8mm tooling v1 (Autodesk Fusion 360 design; units mm, degrees)
Autodesk Fusion 360 part; units mm, degrees
sketch "Sketch1" plane through (0, 0, 0) normal (0, 1, 0) x (1, 0, 0)
  line L0 (0, 0) -> (144, 0)
  line L1 (144, -40) -> (0, -40)
  line L2 (0, -40) -> (0, 0)
  line L3 (0, -20) -> (144, -20)
  line L4 (0, 0) -> (10, 0)
  line L5 (144, 0) -> (140, 0)
  line L6 (10, 0) -> (36, 0)
  line L7 (36, -40) -> (62, -40)
  line L8 (62, 0) -> (88, 0)
  line L9 (88, -40) -> (114, -40)
  line L10 (114, 0) -> (140, 0)
  circle A0 centre (9.5, -30) radius 4
  line L11 (134, -20) -> (144, -20)
  line L12 (144, -40) -> (144, 0)
  line L13 (0, 0) -> (144, 0)
  line L14 (144, 0) -> (144, -5)
  line L15 (144, -5) -> (0, -5)
  line L16 (0, -5) -> (0, 0)
  line L17 (0, -40) -> (5, -40)
  line L18 (5, -40) -> (5, 0)
  line L19 (5, 0) -> (0, 0)
  line L20 (0, 0) -> (0, -40)
  line L21 (144, -40) -> (139, -40)
  line L22 (139, -40) -> (139, 0)
  line L23 (139, 0) -> (144, 0)
  line L24 (144, 0) -> (144, -40)
  circle A1 centre (27.3571, -30) radius 4
  circle A2 centre (45.2143, -30) radius 4
  circle A3 centre (63.0714, -30) radius 4
  circle A4 centre (80.9286, -30) radius 4
  circle A5 centre (98.7857, -30) radius 4
  circle A6 centre (116.6429, -30) radius 4
  circle A7 centre (134.5, -30) radius 4
  circle A8 centre (9.5, -15) radius 4
  circle A9 centre (27.3571, -15) radius 4
  circle A10 centre (45.2143, -15) radius 4
  circle A11 centre (63.0714, -15) radius 4
  circle A12 centre (80.9286, -15) radius 4
  circle A13 centre (98.7857, -15) radius 4
  circle A14 centre (116.6429, -15) radius 4
  circle A15 centre (134.5, -15) radius 4
  dimension "d8" = 8
  dimension "d16" = 5
  dimension "d17" = 5
  dimension "d75" = 125
  dimension "d76" = 15
  constraint horizontal L0
  constraint horizontal L1
  constraint vertical L2
  constraint coincident L0.start L2.end
  constraint midpoint L2 L3.start
  constraint coincident L0 L4.end
  constraint perpendicular L2 L4
  constraint coincident L0 L5.end
  constraint coincident L1 L7.start
  constraint coincident L0 L8.start
  constraint coincident L1 L9.start
  constraint coincident L0 L10.start
  constraint coincident L3 L11.start
  constraint coincident L1 L12.start
  constraint vertical L12
  constraint horizontal L13
  constraint vertical L14
  constraint horizontal L15
  constraint vertical L16
  constraint horizontal L17
  constraint vertical L18
  constraint horizontal L19
  constraint vertical L20
  constraint midpoint L4 L18.end
  constraint horizontal L21
  constraint vertical L22
  constraint horizontal L23
  constraint vertical L24
  measures "d8" diameter of A0
  measures "d16" distance of L0.start L15.end
  measures "d17" distance of L1.start L21.end
extrude "Extrude1" add sketch "Sketch1" along normal blind 5 contours L0 L2 L4 L13 L15 L16 L18 L19 L20 | L0 L4 L6 L8 L10 L13 L15 L18 L22 | L2 L3 L15 L18 L20 | L3 L11 L15 L18 L22 | L1 L2 L3 L17 L18 L20 | L0 L5 L10 L12 L13 L14 L15 L22 L23 L24 | L3 L11 L12 L15 L22 L24 | L1 L3 L7 L9 L11 L18 L22 | L1 L3 L11 L12 L21 L22 L24 | A1 | A2 | A3 | A4 | A5 | A6 | A7 | A8 | A9 | A10 | A11 | A12 | A13 | A14 | A15 makes body 1
fillet "Fillet2" radius 2 2 edges at (72, 5, 40) (72, 0, 40) on bodies 1
sketch "Sketch2" plane through (0, 0, 0) normal (0, -1, 0) x (1, 0, 0)
  line L0 (144, 38) -> (0, 38)
  line L1 (0, 38) -> (0, 0)
  line L2 (0, 0) -> (144, 0)
  line L3 (144, 0) -> (144, 38)
  line L4 (0, 0) -> (144, 0)
  line L5 (144, 0) -> (144, 5)
  line L6 (144, 5) -> (0, 5)
  line L7 (0, 5) -> (0, 0)
  line L8 (0, 0) -> (5, 0)
  line L9 (5, 0) -> (5, 38)
  line L10 (5, 38) -> (0, 38)
  line L11 (0, 38) -> (0, 0)
  line L12 (144, 0) -> (139, 0)
  line L13 (139, 0) -> (139, 38)
  line L14 (139, 38) -> (144, 38)
  line L15 (144, 38) -> (144, 0)
  circle A0 centre (9.5, 30) radius 4
  dimension "d22" = 5
  dimension "d23" = 5
  dimension "d24" = 5
  constraint horizontal L4
  constraint vertical L5
  constraint horizontal L6
  constraint vertical L7
  constraint coincident L1.end L2.start
  constraint horizontal L8
  constraint vertical L9
  constraint horizontal L10
  constraint vertical L11
  constraint horizontal L12
  constraint vertical L13
  constraint horizontal L14
  constraint vertical L15
  measures "d22" distance of L1.end L6.end
  measures "d23" distance of L1.end L8.end
  measures "d24" distance of L2.end L12.end
extrude "Extrude2" add sketch "Sketch2" along normal blind 5 contours L0 L3 L6 L13 L14 L15 | L2 L3 L4 L5 L6 L12 L13 L15 | L0 L1 L6 L9 L10 L11 | L2 L4 L6 L9 L13 | L1 L2 L4 L6 L7 L8 L9 L11 bodies 1
sketch "Sketch3" plane through (0, -5, 0) normal (0, -1, 0) x (1, 0, 0)
  line L0 (139, 38) -> (139, 5)
  line L1 (139, 5) -> (5, 5)
  line L2 (5, 5) -> (5, 38)
  line L3 (0, 38) -> (0, 0)
  line L4 (0, 0) -> (144, 0)
  line L5 (144, 0) -> (144, 38)
  line L6 (72, 0) -> (72, 5)
  line L7 (72, 5) -> (82, 5)
  line L8 (82, 5) -> (82, 0)
  line L9 (82, 0) -> (72, 0)
  line L10 (72, 0) -> (72, 5)
  line L11 (72, 0) -> (62, 0)
  line L12 (62, 0) -> (62, 5)
  line L13 (62, 5) -> (72, 5)
  line L14 (72, 5) -> (72, 0)
  line L15 (5, 5) -> (25, 5)
  line L16 (25, 5) -> (25, 0)
  line L17 (25, 0) -> (5, 0)
  line L18 (5, 0) -> (5, 5)
  line L19 (139, 5) -> (119, 5)
  line L20 (119, 5) -> (119, 0)
  line L21 (119, 0) -> (139, 0)
  line L22 (139, 0) -> (139, 5)
  line L23 (5, 38) -> (0, 38)
  line L24 (144, 38) -> (139, 38)
  dimension "d28" = 10
  dimension "d29" = 10
  dimension "d30" = 20
  dimension "d31" = 20
  constraint midpoint L4 L6.start
  constraint midpoint L1 L6.end
  constraint horizontal L7
  constraint vertical L8
  constraint horizontal L9
  constraint vertical L10
  constraint horizontal L11
  constraint vertical L12
  constraint horizontal L13
  constraint vertical L14
  constraint horizontal L15
  constraint vertical L16
  constraint horizontal L17
  constraint vertical L18
  constraint coincident L1.end L2.start
  constraint horizontal L19
  constraint vertical L20
  constraint horizontal L21
  constraint vertical L22
  constraint coincident L0.end L1.start
  measures "d28" distance of L6.end L7.end
  measures "d29" distance of L6.start L11.end
  measures "d30" distance of L1.end L15.end
  measures "d31" distance of L0.end L19.end
extrude "Extrude3" add sketch "Sketch3" along normal blind 10 contours L1 L4 L19 L20 L21 L22 | L1 L4 L6 L7 L8 L9 L10 L14 | L1 L4 L6 L10 L11 L12 L13 L14 | L1 L4 L15 L16 L17 L18 bodies 1
fillet "Fillet4" radius 10 6 edges at (5, -15, 2.5) (25, -15, 2.5) (62, -15, 2.5) (82, -15, 2.5) (119, -15, 2.5) (139, -15, 2.5) on bodies 1
sketch "Sketch4" plane through (0, 0, 5) normal (0, 0, 1) x (1, 0, 0)
  arc A0 (119, -5) -> (139, -5) centre (129, -5) ccw
  line L0 (139, -5) -> (139, 0)
  line L1 (139, 0) -> (5, 0)
  line L2 (5, 0) -> (5, -5)
  arc A1 (5, -5) -> (25, -5) centre (15, -5) ccw
  line L3 (25, -5) -> (62, -5)
  arc A2 (62, -5) -> (82, -5) centre (72, -5) ccw
  line L4 (82, -5) -> (119, -5)
  line L5 (15, -15) -> (15, 0)
  line L6 (72, -15) -> (72, 0)
  line L7 (129, -15) -> (129, 0)
  line L8 (5, -5) -> (139, -5)
  circle A3 centre (15, -5) radius 1.5
  circle A4 centre (10, -5) radius 1.5
  circle A5 centre (20, -5) radius 1.5
  circle A6 centre (72, -5) radius 1.5
  line L9 (62, -5) -> (82, -5)
  line L10 (62, -5) -> (67, -5)
  line L11 (82, -5) -> (77, -5)
  circle A7 centre (67, -5) radius 1.5
  circle A8 centre (77, -5) radius 1.5
  line L12 (119, -5) -> (139, -5)
  circle A9 centre (129, -5) radius 1.5
  line L13 (119, -5) -> (129, -5)
  circle A10 centre (124, -5) radius 1.5
  line L14 (139, -5) -> (129, -5)
  circle A11 centre (134, -5) radius 1.5
  line L15 (72, -5) -> (72, -15)
  circle A12 centre (72, -10) radius 1.5
  line L16 (15, -15) -> (15, -5)
  circle A13 centre (15, -10) radius 1.5
  line L17 (129, -15) -> (129, -5)
  circle A14 centre (129, -10) radius 1.5
  circle A15 centre (15, 0) radius 1.5
  circle A16 centre (72, 0) radius 1.5
  circle A17 centre (129, 0) radius 1.5
  dimension "d35" = 3
  dimension "d36" = 3
  dimension "d37" = 3
  dimension "d38" = 3
  dimension "d39" = 5
  dimension "d40" = 3
  dimension "d41" = 3
  dimension "d42" = 3
  dimension "d43" = 3
  dimension "d44" = 3
  dimension "d45" = 3
  dimension "d46" = 3
  dimension "d47" = 3
  dimension "d48" = 3
  dimension "d49" = 3
  dimension "d50" = 3
  constraint midpoint A1 L5.start
  constraint coincident L1 L5.end
  constraint midpoint A2 L6.start
  constraint midpoint L1 L6.end
  constraint midpoint A0 L7.start
  constraint coincident L1 L7.end
  constraint vertical L7
  constraint coincident L2.end A1.start
  constraint coincident A0.end L0.start
  constraint concentric A1 A3
  constraint coincident L8 A4.centre
  constraint concentric A2 A6
  constraint coincident L3.end A2.start
  constraint coincident A2.end L4.start
  constraint coincident L9 L10.end
  constraint perpendicular L6 L10
  constraint coincident L10.end A7.centre
  constraint coincident L11.end A8.centre
  constraint coincident A0.start L4.end
  constraint concentric A0 A9
  constraint coincident A0.centre A9.centre
  constraint midpoint L13 A10.centre
  constraint midpoint L14 A11.centre
  constraint coincident A2.centre A6.centre
  constraint midpoint L15 A12.centre
  constraint coincident A1.centre A3.centre
  constraint midpoint L16 A13.centre
  constraint midpoint L17 A14.centre
  constraint coincident L5.end A15.centre
  constraint coincident L6.end A16.centre
  constraint coincident L7.end A17.centre
  measures "d35" diameter of A3
  measures "d36" diameter of A4
  measures "d37" diameter of A5
  measures "d38" diameter of A6
  measures "d39" distance of A2.end L11.end
  measures "d40" diameter of A7
  measures "d41" diameter of A8
  measures "d42" diameter of A9
  measures "d43" diameter of A10
  measures "d44" diameter of A11
  measures "d45" diameter of A12
  measures "d46" diameter of A13
  measures "d47" diameter of A14
  measures "d48" diameter of A15
  measures "d49" diameter of A16
  measures "d50" diameter of A17
extrude "Extrude4" cut sketch "Sketch4" along normal blind 20 contours L8 L12 L13 A10 | L8 L12 L13 A10 | L7 L17 A14 | L7 L17 A14 | L8 L9 L11 A8 | L8 L9 L11 A8 | L8 L12 L14 A11 | L8 L12 L14 A11 | L6 L15 A12 | L6 L15 A12 | L7 L8 L12 A9 L13 | L7 L8 L12 A9 L13 L17 | L1 L7 A17 | L1 A17 | L7 L8 L12 A9 L14 L17 | L8 L9 L10 A7 | L8 L9 L10 A7 | L6 L8 A6 L9 L15 | L6 L8 A6 L9 | L7 L8 L12 A9 L14 | L1 L7 A17 | L8 A5 | L8 A5 | L6 L8 A6 L9 L15 | L6 L8 A6 L9 | L1 L6 A16 | L1 A16 | L5 L16 A13 | L5 L16 A13 | L1 L6 A16 | L8 A4 | L8 A4 | L5 L8 A3 L16 | L5 L8 A3 | L1 L5 A15 | L1 A15 | L1 L5 A15 | L5 L8 A3 L16 | L5 L8 A3 bodies 1
extrude "Extrude5" cut sketch "Sketch4" against normal blind 10 contours L8 L12 L13 A10 | L8 L12 L13 A10 | L7 L17 A14 | L7 L17 A14 | L8 L9 L11 A8 | L8 L9 L11 A8 | L8 L12 L14 A11 | L8 L12 L14 A11 | L6 L15 A12 | L6 L15 A12 | L7 L8 L12 A9 L13 | L7 L8 L12 A9 L13 L17 | L1 L7 A17 | L1 A17 | L7 L8 L12 A9 L14 L17 | L8 L9 L10 A7 | L8 L9 L10 A7 | L6 L8 A6 L9 L15 | L6 L8 A6 L9 | L7 L8 L12 A9 L14 | L1 L7 A17 | L8 A5 | L8 A5 | L6 L8 A6 L9 L15 | L6 L8 A6 L9 | L1 L6 A16 | L1 A16 | L5 L16 A13 | L5 L16 A13 | L1 L6 A16 | L8 A4 | L8 A4 | L5 L8 A3 L16 | L5 L8 A3 | L1 L5 A15 | L1 A15 | L1 L5 A15 | L5 L8 A3 L16 | L5 L8 A3 bodies 1
sketch "Sketch5" plane through (0, 0, 0) normal (0, 0, -1) x (-1, 0, 0)
  arc A0 (-139, -5) -> (-119, -5) centre (-129, -5) ccw
  line L0 (-119, -5) -> (-82, -5)
  arc A1 (-82, -5) -> (-62, -5) centre (-72, -5) ccw
  line L1 (-62, -5) -> (-25, -5)
  arc A2 (-25, -5) -> (-5, -5) centre (-15, -5) ccw
  line L2 (-5, -5) -> (0, -5)
  line L3 (0, -5) -> (0, 5)
  line L4 (0, 5) -> (-144, 5)
  line L5 (-144, 5) -> (-144, -5)
  line L6 (-144, -5) -> (-139, -5)
  circle A3 centre (-15, -10) radius 1.5
  circle A4 centre (-72, -5) radius 1.5
  circle A5 centre (-129, -5) radius 1.5
  circle A6 centre (-15, 0) radius 1.5
  circle A7 centre (-124, -5) radius 1.5
  circle A8 centre (-67, -5) radius 1.5
  circle A9 centre (-10, -5) radius 1.5
  circle A10 centre (-15, -5) radius 1.5
  circle A11 centre (-72, -10) radius 1.5
  circle A12 centre (-129, -10) radius 1.5
  circle A13 centre (-72, 0) radius 1.5
  circle A14 centre (-129, 0) radius 1.5
  circle A15 centre (-134, -5) radius 1.5
  circle A16 centre (-77, -5) radius 1.5
  circle A17 centre (-20, -5) radius 1.5
sketch "Sketch6" plane through (0, 0, 5) normal (0, 0, 1) x (1, 0, 0)
  circle A0 centre (72, 0) radius 3
  circle A1 centre (67, -5) radius 3
  circle A2 centre (77, -5) radius 3
  circle A3 centre (72, -10) radius 3
  circle A4 centre (15, 0) radius 3
  circle A5 centre (10, -5) radius 3
  circle A6 centre (20, -5) radius 3
  circle A7 centre (15, -10) radius 3
  circle A8 centre (129, 0) radius 3
  circle A9 centre (124, -5) radius 3
  circle A10 centre (134, -5) radius 3
  circle A11 centre (129, -10) radius 3
  point P0 (72, 0)
  point P1 (67, -5)
  point P2 (77, -5)
  point P3 (72, -10)
  point P4 (15, 0)
  point P5 (10, -5)
  point P6 (15, -10)
  point P7 (129, 0)
  point P8 (124, -5)
  point P9 (134, -5)
  point P10 (129, -10)
  dimension "d55" = 6
  dimension "d56" = 6
  dimension "d57" = 6
  dimension "d58" = 6
  dimension "d59" = 6
  dimension "d60" = 6
  dimension "d61" = 6
  dimension "d62" = 6
  dimension "d63" = 6
  dimension "d64" = 6
  dimension "d65" = 6
  dimension "d66" = 6
  constraint coincident P0 A0.centre
  constraint coincident P1 A1.centre
  constraint coincident P2 A2.centre
  constraint coincident P3 A3.centre
  constraint coincident P4 A4.centre
  constraint coincident P5 A5.centre
  constraint coincident P6 A7.centre
  constraint coincident P7 A8.centre
  constraint coincident P8 A9.centre
  constraint coincident P9 A10.centre
  constraint coincident P10 A11.centre
  measures "d55" diameter of A0
  measures "d56" diameter of A1
  measures "d57" diameter of A2
  measures "d58" diameter of A3
  measures "d59" diameter of A4
  measures "d60" diameter of A5
  measures "d61" diameter of A6
  measures "d62" diameter of A7
  measures "d63" diameter of A8
  measures "d64" diameter of A9
  measures "d65" diameter of A10
  measures "d66" diameter of A11
chamfer "Chamfer1" distance 3 angle 45 3 edges at (13.6015, -4.4576, 5) (70.6015, -4.4576, 5) (127.6015, -4.4576, 5) on bodies 1
extrude "Extrude6" cut sketch "Sketch6" along normal blind 20 bodies 1
extrude "Extrude7" cut sketch "Sketch6" against normal blind 3.5 bodies 1
fillet "Fillet5" radius 2 3 edges at (15, -15, 5) (72, -15, 5) (129, -15, 5) on bodies 1
extrude "Extrude8" cut sketch "Sketch1" along normal blind 10 contours A1 | A2 | A3 | A4 | A5 | A6 | A7 | A8 | A9 | A10 | A11 | A12 | A13 | A14 | A15 bodies 1
fillet "Fillet7" radius 3 16 edges at (130.7707, 5, 28.5535) (130.7707, 5, 13.5535) (112.9135, 5, 28.5535) (112.9135, 5, 13.5535) (95.0564, 5, 28.5535) (95.0564, 5, 13.5535) (77.1993, 5, 28.5535) (77.1993, 5, 13.5535) (59.3421, 5, 28.5535) (59.3421, 5, 13.5535) (41.485, 5, 28.5535) (41.485, 5, 13.5535) (23.6278, 5, 28.5535) (23.6278, 5, 13.5535) (5.7707, 5, 13.5535) (5.7707, 5, 28.5535) on bodies 1
sketch "Sketch7" plane through (0, 0, 0) normal (0, -1, 0) x (1, 0, 0)
  circle A0 centre (9.5, 30) radius 4
  arc A1 (132, 11.8775) -> (132, 18.1225) centre (134.5, 15) ccw
  line L0 (132, 11.8775) -> (132, 5)
  line L1 (132, 5) -> (139, 5)
  line L2 (139, 5) -> (139, 38)
  line L3 (139, 38) -> (5, 38)
  line L4 (5, 38) -> (5, 5)
  line L5 (5, 5) -> (12, 5)
  line L6 (12, 5) -> (12, 11.8775)
  arc A2 (12, 18.1225) -> (12, 11.8775) centre (9.5, 15) ccw
  line L7 (12, 18.1225) -> (12, 25)
  line L8 (12, 25) -> (18, 25)
  line L9 (18, 25) -> (18, 5)
  line L10 (18, 5) -> (69, 5)
  line L11 (69, 5) -> (69, 25)
  line L12 (69, 25) -> (75, 25)
  line L13 (75, 25) -> (75, 5)
  line L14 (75, 5) -> (126, 5)
  line L15 (126, 5) -> (126, 25)
  line L16 (126, 25) -> (132, 25)
  line L17 (132, 25) -> (132, 18.1225)
  circle A3 centre (80.9286, 15) radius 4
  circle A4 centre (134.5, 30) radius 4
  circle A5 centre (63.0714, 30) radius 4
  circle A6 centre (45.2143, 30) radius 4
  circle A7 centre (116.6429, 30) radius 4
  circle A8 centre (98.7857, 15) radius 4
  circle A9 centre (27.3571, 15) radius 4
  circle A10 centre (63.0714, 15) radius 4
  circle A11 centre (80.9286, 30) radius 4
  circle A12 centre (27.3571, 30) radius 4
  circle A13 centre (98.7857, 30) radius 4
  circle A14 centre (116.6429, 15) radius 4
  circle A15 centre (45.2143, 15) radius 4
  line L18 (27.3571, 30) -> (45.2143, 30)
  line L19 (45.2143, 30) -> (45.2143, 15)
  line L20 (45.2143, 15) -> (27.3571, 15)
  line L21 (27.3571, 15) -> (27.3571, 30)
  line L22 (36.2857, 30) -> (34.2857, 30)
  line L23 (34.2857, 30) -> (38.2857, 30)
  line L24 (38.2857, 30) -> (38.2857, 15)
  line L25 (38.2857, 15) -> (34.2857, 15)
  line L26 (34.2857, 15) -> (34.2857, 30)
  line L27 (34.2857, 30) -> (38.2857, 30)
  line L28 (38.2857, 30) -> (38.2857, 5)
  line L29 (38.2857, 5) -> (34.2857, 5)
  line L30 (34.2857, 5) -> (34.2857, 30)
  dimension "d83" = 4
  dimension "d84" = 4
  constraint coincident A12.centre L18.start
  constraint coincident A6.centre L18.end
  constraint coincident A15.centre L19.end
  constraint coincident A9.centre L20.end
  constraint midpoint L18 L22.start
  constraint horizontal L23
  constraint vertical L24
  constraint horizontal L25
  constraint vertical L26
  constraint horizontal L27
  constraint vertical L28
  constraint horizontal L29
  constraint vertical L30
  measures "d83" distance of L22.end L23.end
  measures "d84" distance of L22.end L23.end
extrude "Extrude9" add sketch "Sketch7" along normal blind 16 contours L10 L20 L25 L28 L29 L30 | L18 L20 L22 L23 L24 L25 L26 L27 L28 L30 bodies 1
sketch "Sketch8" plane through (0, -5, 0) normal (0, -1, 0) x (1, 0, 0)
  line L0 (139, 3) -> (139, 0)
  line L1 (139, 0) -> (144, 0)
  line L2 (144, 0) -> (144, 38)
  line L3 (144, 38) -> (139, 38)
  line L4 (139, 38) -> (139, 5)
  line L5 (139, 5) -> (137, 5)
  arc A0 (139, 3) -> (137, 5) centre (137, 3) ccw
  line L6 (139, 38) -> (144, 38)
  line L7 (144, 38) -> (144, 0)
  line L8 (144, 0) -> (139, 0)
  line L9 (139, 0) -> (139, 38)
  constraint horizontal L6
  constraint vertical L7
  constraint horizontal L8
  constraint vertical L9
  constraint coincident L1.end L2.start
  constraint coincident L3.end L4.start
extrude "Extrude10" add sketch "Sketch8" against normal blind 5 contours L0 L1 L2 L3 L4 L6 L7 L8 L9 bodies 1
sketch "Sketch9" plane through (144, 0, 0) normal (1, 0, 0) x (0, 0, -1)
  arc A0 (-40, 2) -> (-38, 0) centre (-38, 2) ccw
  line L0 (-38, 0) -> (-38, -5)
  line L1 (0, -5) -> (0, 5)
  line L2 (0, 5) -> (-38, 5)
  arc A1 (-38, 5) -> (-40, 3) centre (-38, 3) ccw
  line L3 (-40, 3) -> (-40, 2)
  line L4 (-38, -5) -> (0, -5)
sketch "Sketch10" plane through (0, 0, 5) normal (0, 0, -1) x (-1, 0, 0)
  line L0 (-34.2857, -5) -> (-38.2857, -5)
  line L1 (-38.2857, -5) -> (-38.2857, -16)
  line L2 (-34.2857, -16) -> (-34.2857, -5)
  line L3 (-38.2857, -16) -> (-34.2857, -16)
  line L4 (-34.2857, -16) -> (-34.2857, -5)
  line L5 (-34.2857, -5) -> (-38.2857, -5)
  line L6 (-38.2857, -5) -> (-38.2857, -16)
  line L7 (-38.2857, -16) -> (-34.2857, -16)
  constraint horizontal L3
  constraint vertical L4
  constraint horizontal L5
  constraint vertical L6
  constraint coincident L0.start L2.end
  constraint coincident L1.end L3.start
extrude "Extrude11" add sketch "Sketch10" along normal blind 5 bodies 1
move_face "OffsetFaces1" offset -1 1 faces at (36.9524, -16, 20) on bodies 1
move_face "OffsetFaces2" offset -10 1 faces at (36.9524, -15, 20) on bodies 1
copy_body "CopyPasteBodies1" bodies 1 makes body 2
move_body "Move1" bodies 2 to x (1, 0, 0) y (0, 1, 0) z (0, 0, 1) at (0, -10, 0)
move_body "Move2" bodies 2 to x (-1, 0, 0) y (0, -1, 0) z (0, 0, 1) at (288, -30, 0)
move_body "Move3" bodies 2 to x (1, 0, 0) y (0, 1, 0) z (0, 0, 1) at (-144, 10, 0)
sketch "Sketch11" plane through (0, -5, 0) normal (0, 1, 0) x (-1, 0, 0)
  line L0 (-109.7143, 5) -> (-121, 5)
  arc A0 (-119, 3) -> (-121, 5) centre (-121, 3) ccw
  line L1 (-119, 3) -> (-119, 0)
  line L2 (-119, 0) -> (-82, 0)
  line L3 (-82, 0) -> (-82, 3)
  arc A1 (-80, 5) -> (-82, 3) centre (-80, 3) ccw
  line L4 (-80, 5) -> (-105.7143, 5)
  line L5 (-105.7143, 5) -> (-105.7143, 30)
  line L6 (-105.7143, 30) -> (-109.7143, 30)
  line L7 (-109.7143, 30) -> (-109.7143, 5)
  line L8 (-105.7143, 5) -> (-109.7143, 5)
  line L9 (-109.7143, 5) -> (-109.7143, 30)
  line L10 (-109.7143, 30) -> (-105.7143, 30)
  line L11 (-105.7143, 30) -> (-105.7143, 5)
  constraint horizontal L8
  constraint vertical L9
  constraint horizontal L10
  constraint vertical L11
  constraint coincident L6.end L7.start
  constraint coincident L4.end L5.start
extrude "Extrude12" add sketch "Sketch11" along normal blind 10 contours L5 L6 L7 L8 L9 L10 L11 bodies 1 2
sketch "Sketch12" plane through (0, -5, 0) normal (0, -1, 0) x (1, 0, 0)
  line L0 (34.2857, 5) -> (38.2857, 5)
  line L1 (38.2857, 5) -> (38.2857, 30)
  line L2 (38.2857, 30) -> (34.2857, 30)
  line L3 (34.2857, 30) -> (34.2857, 5)
  line L4 (34.2857, 30) -> (38.2857, 30)
  line L5 (38.2857, 30) -> (38.2857, 5)
  line L6 (38.2857, 5) -> (34.2857, 5)
  line L7 (34.2857, 5) -> (34.2857, 30)
  constraint horizontal L4
  constraint vertical L5
  constraint horizontal L6
  constraint vertical L7
  constraint coincident L0.end L1.start
  constraint coincident L2.end L3.start
extrude "Extrude13" add sketch "Sketch12" along normal blind 10 bodies 1
